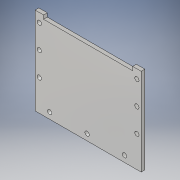
# Autodesk Inventor part: КВ33.000.103 - Стенка тонкая
Saved by Autodesk Inventor 2019 (Build 230136000, 136)
## iProperties
Created: 2021-03-13
Part Number: КВ33.000.103 - Стенка тонкая
Material: Generic
Document SubType Name: Modeling
Designer: Петров Иван
Density: 1 g/cm^3
Appearance: Aluminum - Dark
Sheet Metal Rule: Default_mm
Author: Петров Иван
Autodesk Inventor part; units mm, degrees
ref_plane "YZ Plane" through (0, 0, 0) normal (1, 0, 0) x (0, 1, 0)
ref_plane "XZ Plane" through (0, 0, 0) normal (0, 1, 0) x (-1, 0, 0)
ref_plane "XY Plane" through (0, 0, 0) normal (0, 0, 1) x (1, 0, 0)
sketch "Sketch1" plane through (0, 0, 0) normal (0, 0, 1) x (1, 0, 0)
  circle A0 centre (81.6123, 24.8914) radius 1.75 projected
  circle A1 centre (81.6123, 43.8914) radius 1.75 projected
  circle A2 centre (81.6123, 62.8914) radius 1.75 projected
  line L0 (78.2246, 67) -> (71.4493, 67) projected
  line L1 (71.4493, 46.4435) -> (71.4493, 20) projected
  line L2 (80, 20) -> (71.4493, 20) projected
  line L3 (80, 10) -> (80, 20) projected
  line L4 (85, 10) -> (80, 10) projected
  line L5 (85, 10) -> (85, 70) projected
  line L6 (85, 70) -> (78.2246, 70) projected
  line L7 (78.2246, 70) -> (78.2246, 67) projected
  circle A3 centre (3.3877, 24.8914) radius 1.75 projected
  circle A4 centre (3.3877, 43.8914) radius 1.75 projected
  circle A5 centre (3.3877, 62.8914) radius 1.75 projected
  line L8 (13.5507, 67) -> (6.7754, 67) projected
  line L9 (6.7754, 67) -> (6.7754, 70) projected
  line L10 (0, 70) -> (6.7754, 70) projected
  line L11 (0, 10) -> (0, 70) projected
  line L12 (0, 10) -> (5, 10) projected
  line L13 (5, 20) -> (5, 10) projected
  line L14 (5, 20) -> (13.5507, 20) projected
  line L15 (13.5507, 50.4435) -> (13.5507, 67) projected
  circle A6 centre (71.6772, 5) radius 1.75 projected
  circle A7 centre (56.6772, 5) radius 1.75 projected
  circle A8 centre (26.6772, 5) radius 1.75 projected
  circle A9 centre (11.6772, 5) radius 1.75 projected
  circle A10 centre (41.6772, 5) radius 1.75 projected
  line L16 (0, 0) -> (85, 0) projected
  line L17 (85, 0) -> (85, 10) projected
  line L18 (80, 10) -> (85, 10) projected
  line L19 (80, 10) -> (80, 20) projected
  line L20 (5, 20) -> (80, 20) projected
  line L21 (5, 10) -> (5, 20) projected
  line L22 (0, 10) -> (5, 10) projected
  line L23 (0, 0) -> (0, 10) projected
  line L24 (13.5507, 67) -> (71.4493, 67)
  line L25 (71.4493, 50.4435) -> (79.4493, 50.4435) projected
  line L26 (79.4493, 50.4435) -> (79.4493, 46.4435) projected
  line L27 (79.4493, 46.4435) -> (71.4493, 46.4435) projected
  line L28 (71.4493, 67) -> (71.4493, 50.4435) projected
  line L29 (5.5507, 50.4435) -> (13.5507, 50.4435) projected
  line L30 (13.5507, 20) -> (13.5507, 46.4435) projected
  line L31 (13.5507, 46.4435) -> (5.5507, 46.4435) projected
  line L32 (5.5507, 46.4435) -> (5.5507, 50.4435) projected
  constraints: 2 end point, 1 collinear
extrude "Extrusion1" add sketch "Sketch1" along normal blind 3 contours L7 L6 L5 L4 L3 L2 L1 L27 L26 L25 L28 L0 | L28 L25 L26 L27 L1 L20 L30 L31 L32 L29 L15 L24 | L15 L29 L32 L31 L30 L14 L13 L12 L11 L10 L9 L8 | L17 L16 L23 L12 L13 L14 L20 L2 L3 L4 | A7 | A8
equation "\"BendRadius\" = Thickness"
equation "\"BendReliefWidth\" = Thickness"
equation "\"BendReliefDepth\" = 0.5 * Thickness"
equation "\"CornerReliefSize\" = 4 * Thickness"
equation "\"MinimumRemnant\" = 2 * Thickness"
equation "\"TransitionRadius\" = BendRadius"
equation "\"JacobiRadiusSize\" = BendRadius"
equation "\"GapSize\" = Thickness"
equation "\"Thickness\" = 3"
body "Solid1"
